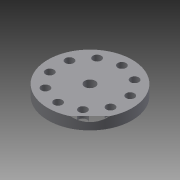
# Autodesk Inventor part: EncoderWheel2
Saved by Autodesk Inventor 2014 (Build 180170000, 170)
## iProperties
Created: 2013-05-31
Part Number: EncoderWheel2
Material: Generisch
Document SubType Name: Modeling
Designer: hanse
Density: 1 g/cm^3
Appearance: Vorgabe
Author: hanse
Autodesk Inventor part; units mm, degrees
ref_plane "YZ Plane" through (0, 0, 0) normal (1, 0, 0) x (0, 1, 0)
ref_plane "XZ Plane" through (0, 0, 0) normal (0, 1, 0) x (-1, 0, 0)
ref_plane "XY Plane" through (0, 0, 0) normal (0, 0, 1) x (1, 0, 0)
sketch "Skizze3" plane through (0, 0, 0) normal (0, 0, 1) x (1, 0, 0)
  circle A0 centre (0, 0) radius 7.5
  dimension "d13" = 15
  constraints: 1 centre point, 1 coincident
  measures "d13" diameter of A0
extrude "Extrusion3" add sketch "Skizze3" along normal blind 1.9
sketch "Skizze4" plane through (0, 0, 1.9) normal (0, 0, 1) x (1, 0, 0)
  circle A0 centre (0, 0) radius 7.5 projected
  circle A1 centre (0, 5.7) radius 0.75
  line L0 (0, 5.7) -> (0, 7.5)
  dimension "d17" = 1.5
  dimension "d26" = 1.8
  constraints: 2 end point, 1 centre point, 1 vertical, 1 vertical alignment, 1 other
  measures "d17" diameter of A1
  measures "d26" distance of L0.end L0.start
extrude "Extrusion4" cut sketch "Skizze4" against normal through all contours A1
pattern_circular "Runde Anordnung1" count 10 over 360 about axis through (0, 0, -10) along (0, 0, 1) of "Extrusion4"
sketch "Skizze5" plane through (0, 0, 1.9) normal (0, 0, 1) x (1, 0, 0)
  circle A0 centre (0, 0) radius 7.5 projected
  circle A1 centre (0, 0) radius 0.95
  dimension "d23" = 1.9
  constraints: 1 centre point, 1 coincident
  measures "d23" diameter of A1
extrude "Extrusion5" cut sketch "Skizze5" against normal through all contours A1
